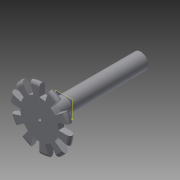
# Autodesk Inventor part: Part1
Saved by Autodesk Inventor 2015 (Build 190159000, 159)
## iProperties
Created: 2015-12-10
Part Number: Part1
Material: Generic
Document SubType Name: Modeling
Designer: Ross
Density: 1 g/cm^3
Appearance: Default
Author: Ross
Autodesk Inventor part; units mm, degrees
ref_plane "YZ Plane" through (0, 0, 0) normal (1, 0, 0) x (0, 1, 0)
ref_plane "XZ Plane" through (0, 0, 0) normal (0, 1, 0) x (-1, 0, 0)
ref_plane "XY Plane" through (0, 0, 0) normal (0, 0, 1) x (1, 0, 0)
sketch "Sketch1" plane through (0, 0, 0) normal (0, 1, 0) x (-1, 0, 0)
  line L0 (0, 0) -> (16, 0)
  arc A0 (16, 0) -> (15.2169, 4.9443) centre (0, 0) ccw
  line L1 (0, 0) -> (15.2169, 4.9443) construction
  line L2 (0, 0) -> (16, 0) construction
  line L3 (15.2169, 4.9443) -> (0, 0)
  arc A1 (16, 0) -> (15.2169, 4.9443) centre (0, 0) ccw
  line L4 (16, 0) -> (0, 0)
  line L5 (0, 0) -> (15.2169, 4.9443)
  dimension "d1" = 18
  constraints: 12 end point, 4 point on circle, 2 centre point, 2 coincident, 2 horizontal, 1 collinear
  measures "d1" angle of L2 L1
extrude "Extrusion1" add sketch "Sketch1" along normal blind 3
fillet "Fillet1" radius 2 2 edges at (-15.803, 0, 2.503) (-15.803, 3, 2.503)
pattern_circular "Circular Pattern1" count 10 over 360 about axis through (0, -10, 0) along (0, 1, 0) of "Extrusion1"
sketch "Sketch2" plane through (0, 0, 0) normal (0, 1, 0) x (-1, 0, 0)
  circle A0 centre (0, 0) radius 10
  dimension "d8" = 20
  constraints: 1 centre point, 1 coincident
  measures "d8" diameter of A0
extrude "Extrusion2" add sketch "Sketch2" along normal blind 3
fillet "Fillet2" radius 2 7 edges at (15.803, 3, -2.503) (14.2561, 3, 7.2638) (7.2638, 3, 14.2561) (-2.503, 3, 15.803) (-7.2638, 3, -14.2561) (2.503, 3, -15.803) (11.3137, 3, -11.3137)
fillet "Fillet3" radius 2 9 edges at (-2.503, 0, 15.803) (-11.3137, 0, 11.3137) (7.2638, 0, 14.2561) (14.2561, 0, 7.2638) (15.803, 0, -2.503) (11.3137, 0, -11.3137) (2.503, 0, -15.803) (-14.2561, 0, -7.2638) (-7.2638, 0, -14.2561)
fillet "Fillet4" radius 2 2 edges at (-11.3137, 3, 11.3137) (-14.2561, 3, -7.2638)
sketch "Sketch3" plane through (0, 0, 0) normal (0, -1, 0) x (1, 0, 0)
  circle A0 centre (0, 0) radius 0.9
  dimension "d14" = 1.8
  constraints: 1 centre point, 1 coincident
  measures "d14" diameter of A0
extrude "Extrusion3" cut sketch "Sketch3" against normal blind 8
sketch "Sketch4" plane through (0, 3, 0) normal (0, 1, 0) x (1, 0, 0)
  circle A0 centre (0, 0) radius 4.1
  dimension "d17" = 8.2
  constraints: 1 centre point, 1 coincident
  measures "d17" diameter of A0
extrude "Extrusion4" add sketch "Sketch4" along normal blind 40
sketch "Sketch5" plane through (0, 43, 0) normal (0, 1, 0) x (1, 0, 0)
  circle A0 centre (0, 0) radius 4.1
  dimension "d20" = 8.2
  constraints: 1 centre point, 1 coincident
  measures "d20" diameter of A0
extrude "Extrusion5" add sketch "Sketch5" along normal blind 10
ref_plane "Work Plane1" through (0, 13, 0) normal (0, 1, 0) x (1, 0, 0)
sketch "Sketch6" plane through (0, 53, 0) normal (0, 1, 0) x (1, 0, 0)
  circle A0 centre (0, 0) radius 2.6
  dimension "d24" = 5.2
  constraints: 1 centre point, 1 coincident
  measures "d24" diameter of A0
extrude "Extrusion6" cut sketch "Sketch6" against normal blind 40
body "Solid1"
